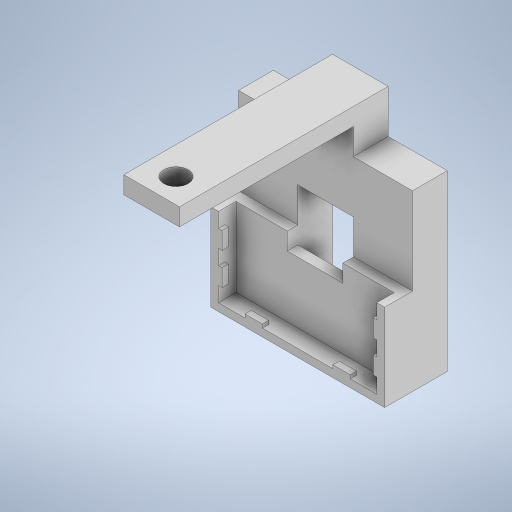
# Autodesk Inventor part: sensor mount
Saved by Autodesk Inventor 2023 (Build 270158000, 158)
## iProperties
Created: 2023-02-01
Part Number: sensor mount
Material: Generic
Document SubType Name: Modeling
Designer: royal
Density: 1 g/cm^3
Appearance: Default
Author: royal
Autodesk Inventor part; units mm, degrees
ref_plane "YZ Plane" through (0, 0, 0) normal (1, 0, 0) x (0, 1, 0)
ref_plane "XZ Plane" through (0, 0, 0) normal (0, 1, 0) x (-1, 0, 0)
ref_plane "XY Plane" through (0, 0, 0) normal (0, 0, 1) x (1, 0, 0)
sketch "Sketch1" plane through (0, 0, 0) normal (0, 0, 1) x (1, 0, 0)
  line L0 (-25, 12.5) -> (25, 12.5)
  line L1 (25, 12.5) -> (25, -12.5)
  line L2 (25, -12.5) -> (-25, -12.5)
  line L3 (-25, -12.5) -> (-25, 12.5)
  line L4 (-25, 12.5) -> (25, -12.5) construction
  line L5 (25, 12.5) -> (-25, -12.5) construction
  line L6 (-25, 12.5) -> (25, 12.5) construction
  point P0 (0, 0)
  dimension "d0" = 50
  dimension "d1" = 0
  dimension "d2" = 25
  constraints: 14 end point, 2 horizontal, 2 midpoint, 2 parallel, 1 collinear, 1 perpendicular
  measures "d0" distance of L0.start L0.end
  measures "d1" distance between parallel lines of L0 L6
  measures "d2" distance of L0.end L1.end
extrude "Extrusion1" add sketch "Sketch1" along normal blind 3
sketch "Sketch2" plane through (0, 0, 3) normal (0, 0, 1) x (1, 0, 0)
  line L0 (-22.75, -10.25) -> (22.75, -10.25)
  line L1 (22.75, -10.25) -> (22.75, 10.25)
  line L2 (22.75, 10.25) -> (-22.75, 10.25)
  line L3 (-22.75, 10.25) -> (-22.75, -10.25)
  line L4 (-22.75, -10.25) -> (22.75, 10.25) construction
  line L5 (22.75, -10.25) -> (-22.75, 10.25) construction
  line L6 (-22.75, -10.25) -> (22.75, -10.25) construction
  line L7 (25, 12.5) -> (-25, 12.5) projected
  line L8 (-25, -12.5) -> (25, -12.5) projected
  line L9 (25, 12.5) -> (25, -12.5)
  line L10 (25, -12.5) -> (-25, -12.5)
  line L11 (-25, -12.5) -> (-25, 12.5)
  line L12 (-22.75, 10.25) -> (-22.75, 12.5)
  line L13 (22.75, 10.25) -> (22.75, 12.5)
  line L14 (-25, 12.5) -> (-22.75, 12.5)
  line L15 (22.75, 12.5) -> (25, 12.5)
  point P0 (0, 0)
  dimension "d5" = 45.5
  dimension "d6" = 0
  dimension "d7" = 20.5
  constraints: 28 end point, 6 perpendicular, 5 parallel, 4 horizontal, 2 midpoint, 1 collinear
  measures "d5" distance of L0.start L0.end
  measures "d6" distance between parallel lines of L0 L6
  measures "d7" distance of L1.end L0.end
extrude "Extrusion2" add sketch "Sketch2" along normal blind 5 contours L0 L1 L13 L7 L9 L8 L11 L12 L3
sketch "Sketch3" plane through (-22.75, -10.25, 3) normal (1, 0, 0) x (0, 0, -1)
  line L0 (-5, 0) -> (-5, 22.75) projected
  line L1 (-3.2, 18.5) -> (-5, 18.5)
  line L2 (-5, 18.5) -> (-5, 13.5)
  line L3 (-5, 13.5) -> (-3.2, 13.5)
  line L4 (-3.2, 13.5) -> (-3.2, 18.5)
  line L5 (-5, 4.25) -> (-3.2, 4.25)
  line L6 (-3.2, 4.25) -> (-3.2, 9.25)
  line L7 (-3.2, 9.25) -> (-5, 9.25)
  line L8 (-5, 9.25) -> (-5, 4.25)
  point P0 (3, 10.25)
  point P1 (-5, 9.25)
  point P2 (-5, 4.25)
  dimension "d10" = 5
  dimension "d11" = 5
  dimension "d28" = 1.8
  constraints: 16 end point, 4 parallel, 3 point on line, 2 horizontal, 2 perpendicular
  measures "d10" distance of L2.end L1.end
  measures "d11" distance of L6.end L5.end
  measures "d28" distance of L2.end L3.end
extrude "Extrusion3" add sketch "Sketch3" along normal blind 1
sketch "Sketch4" plane through (22.75, -10.25, 3) normal (-1, 0, 0) x (0, 0, 1)
  line L0 (5, 18.5) -> (5, 13.5) projected
  line L1 (3.2, 13.5) -> (3.2, 18.5) projected
  line L2 (5, 18.5) -> (3.2, 18.5)
  line L3 (3.2, 18.5) -> (3.2, 13.5)
  line L4 (3.2, 13.5) -> (5, 13.5)
  line L5 (5, 13.5) -> (5, 18.5)
  line L6 (5, 9.25) -> (5, 13.5) projected
  line L7 (3.2, 9.25) -> (3.2, 4.25) projected
  line L8 (5, 9.25) -> (3.2, 9.25)
  line L9 (3.2, 9.25) -> (3.2, 4.25)
  line L10 (3.2, 4.25) -> (5, 4.25)
  line L11 (5, 4.25) -> (5, 9.25)
  point P0 (-3, 10.25)
  constraints: 16 end point, 4 parallel, 2 horizontal, 2 perpendicular
extrude "Extrusion4" add sketch "Sketch4" along normal blind 1
sketch "Sketch5" plane through (-22.75, -10.25, 3) normal (0, 1, 0) x (1, 0, 0)
  line L0 (45.5, -5) -> (0, -5) projected
  line L1 (7.625, -5) -> (12.625, -5)
  line L2 (12.625, -5) -> (12.625, -3.2)
  line L3 (12.625, -3.2) -> (7.625, -3.2)
  line L4 (7.625, -3.2) -> (7.625, -5)
  line L5 (32.875, -5) -> (37.875, -5)
  line L6 (37.875, -5) -> (37.875, -3.2)
  line L7 (37.875, -3.2) -> (32.875, -3.2)
  line L8 (32.875, -3.2) -> (32.875, -5)
  point P0 (22.75, 3)
  dimension "d31" = 5
  dimension "d32" = 1.8
  dimension "d33" = 5
  dimension "d34" = 1.8
  constraints: 16 end point, 4 parallel, 2 horizontal, 2 perpendicular, 2 point on line
  measures "d31" distance of L3.end L2.end
  measures "d32" distance of L2.end L1.end
  measures "d33" distance of L7.end L6.end
  measures "d34" distance of L6.end L5.end
extrude "Extrusion5" add sketch "Sketch5" along normal blind 1
sketch "Sketch6" plane through (0, 0, 0) normal (0, 0, -1) x (-1, 0, 0)
  line L0 (25, -12.5) -> (-25, -12.5) projected
  line L1 (-8, -12.5) -> (-25, -12.5)
  line L2 (-25, -12.5) -> (-25, 37.5)
  line L3 (-25, 37.5) -> (-8, 37.5)
  line L4 (-8, 37.5) -> (-8, -12.5)
  line L5 (8, -12.5) -> (25, -12.5)
  line L6 (25, -12.5) -> (25, 37.5)
  line L7 (25, 37.5) -> (8, 37.5)
  line L8 (8, 37.5) -> (8, -12.5)
  line L9 (-8, 50) -> (-8, 22.5)
  line L10 (-8, 22.5) -> (8, 22.5)
  line L11 (-8, 50) -> (8, 50)
  line L12 (-8, 50) -> (8, 50) construction
  line L13 (8, 50) -> (8, 37.5)
  point P0 (0, 0)
  point P1 (-25, -12.5)
  point P2 (25, -12.5)
  point P3 (8, 50)
  dimension "d41" = 17
  dimension "d42" = 50
  dimension "d43" = 17
  dimension "d44" = 50
  dimension "d47" = 16
  dimension "d49" = 0
  constraints: 26 end point, 4 parallel, 3 horizontal, 3 perpendicular, 1 collinear
  measures "d41" distance of L2.end L3.end
  measures "d42" distance of L1.end L2.end
  measures "d43" distance of L7.end L6.end
  measures "d44" distance of L6.end L5.end
  measures "d47" distance of L10.end L9.end
  measures "d49" distance between parallel lines of L11 L12
extrude "Extrusion6" add sketch "Sketch6" along normal blind 10 contours L0 L8 L7 L6 | L0 L2 L3 L4 | L10 L4 L9 L11 L13 L8
sketch "Sketch7" plane through (0, 0, 3) normal (0, 0, 1) x (1, 0, 0)
  line L0 (22.75, 12.5) -> (-22.75, 12.5) projected
  line L1 (-8, 12.5) -> (8, 12.5)
  line L2 (8, 12.5) -> (8, 7.5)
  line L3 (8, 7.5) -> (-8, 7.5)
  line L4 (-8, 7.5) -> (-8, 12.5)
  point P0 (0, 0)
  dimension "d35" = 16
  dimension "d36" = 5
  constraints: 8 end point, 2 parallel, 1 horizontal, 1 perpendicular, 1 point on line
  measures "d35" distance of L2.end L3.end
  measures "d36" distance of L1.end L2.end
extrude "Extrusion7" cut sketch "Sketch7" against normal through all
sketch "Sketch18" plane through (-8, 50, 0) normal (0, 1, 0) x (1, 0, 0)
  line L0 (0, 0) -> (16, 0) projected
  line L1 (0, 0) -> (16, 0)
  line L2 (16, 0) -> (16, -50)
  line L3 (16, -50) -> (0, -50)
  line L4 (0, -50) -> (0, 0)
  line L5 (16, 0) -> (16, 10) projected
  circle A0 centre (8, -43) radius 3.5
  point P0 (8, 0)
  point P1 (8, 0)
  dimension "d86" = 50
  dimension "d87" = 7
  dimension "d88" = 7
  constraints: 8 end point, 2 parallel, 1 centre point, 1 collinear, 1 horizontal, 1 midpoint, 1 perpendicular, 1 vertical alignment
  measures "d86" distance of L3.end L0.start
  measures "d87" diameter of A0
  measures "d88" distance from line of L3 A0.centre
extrude "Extrusion15" add sketch "Sketch18" against normal blind 5
body "Solid1"
